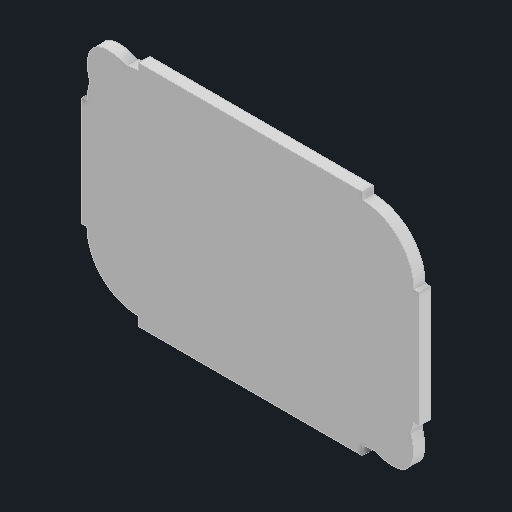
# Autodesk Inventor part: CalibrationTarget
Saved by Autodesk Inventor 2026 (Build 300175050, 175E)
## iProperties
Created: 2024-11-18
Part Number: CalibrationTarget
Material: Generisch
Document SubType Name: Modeling
Designer: neuhau0004
Density: 1 g/cm^3
Appearance: Vorgabe
Author: neuhau0004
Autodesk Inventor part; units mm, degrees
ref_plane "YZ Plane" through (0, 0, 0) normal (1, 0, 0) x (0, 1, 0)
ref_plane "XZ Plane" through (0, 0, 0) normal (0, 1, 0) x (-1, 0, 0)
ref_plane "XY Plane" through (0, 0, 0) normal (0, 0, 1) x (1, 0, 0)
sketch "Skizze1" plane through (0, 0, 0) normal (0, 0, 1) x (1, 0, 0)
  line L0 (-62.3, -42.85) -> (62.3, -42.85)
  line L1 (62.3, -42.85) -> (62.3, 42.85)
  line L2 (62.3, 42.85) -> (-62.3, 42.85)
  line L3 (-62.3, 42.85) -> (-62.3, -42.85)
  line L4 (-62.3, -42.85) -> (62.3, 42.85) construction
  line L5 (62.3, -42.85) -> (-62.3, 42.85) construction
  line L6 (-62, 42.85) -> (62, 42.85)
  line L7 (64, 40.85) -> (64, -40.85)
  line L8 (62, -42.85) -> (-62, -42.85)
  line L9 (-64, -40.85) -> (-64, 40.85)
  line L10 (-64, 42.85) -> (64, -42.85) construction
  line L11 (64, 42.85) -> (-64, -42.85) construction
  circle A0 centre (-40, 19.85) radius 18.45
  circle A1 centre (0, 19.85) radius 18.45
  circle A2 centre (40, 19.85) radius 18.45
  circle A3 centre (-40, -19.15) radius 18.45
  circle A4 centre (0, -19.15) radius 18.45
  circle A5 centre (40, -19.15) radius 18.45
  arc A6 (64, 40.85) -> (62, 42.85) centre (62, 40.85) ccw
  arc A7 (62, -42.85) -> (64, -40.85) centre (62, -40.85) ccw
  arc A8 (-64, -40.85) -> (-62, -42.85) centre (-62, -40.85) ccw
  arc A9 (-62, 42.85) -> (-64, 40.85) centre (-62, 40.85) ccw
  line L12 (-60.3, 40.85) -> (60.3, 40.85)
  line L13 (60.3, 40.85) -> (60.3, -40.85)
  line L14 (60.3, -40.85) -> (-60.3, -40.85)
  line L15 (-60.3, -40.85) -> (-60.3, 40.85)
  line L16 (-60.3, 40.85) -> (60.3, -40.85) construction
  line L17 (60.3, 40.85) -> (-60.3, -40.85) construction
  ellipse E0 centre (40, 19.85) end of major axis (24, 37.55) minor radius 11.9962
  ellipse E1 centre (0, 19.85) end of major axis (-16, 37.55) minor radius 11.9962
  ellipse E2 centre (-40, 19.85) end of major axis (-56, 37.55) minor radius 11.9962
  ellipse E3 centre (40, -19.15) end of major axis (24, -1.45) minor radius 11.9962
  ellipse E4 centre (0, -19.15) end of major axis (-16, -1.45) minor radius 11.9962
  ellipse E5 centre (-40, -19.15) end of major axis (-56, -1.45) minor radius 11.9962
  line L18 (-40, 40.85) -> (-60.3, 40.85)
  line L19 (-60.3, 40.85) -> (-60.3, 19.85)
  line L20 (-58.45, 19.85) -> (-60.3, 19.85)
  line L21 (-58.45, -19.15) -> (-60.3, -19.15)
  line L22 (-60.3, -40.85) -> (-60.3, -19.15)
  line L23 (-40, -37.6) -> (-40, -40.85)
  line L24 (-60.3, -40.85) -> (-40, -40.85)
  arc A10 (-40, 38.3) -> (-58.45, 19.85) centre (-40, 19.85) ccw
  line L25 (-40, 40.85) -> (-40, 38.3)
  line L26 (40, 38.3) -> (40, 40.85)
  line L27 (58.45, 19.85) -> (60.3, 19.85)
  line L28 (58.45, -19.15) -> (60.3, -19.15)
  line L29 (40, -37.6) -> (40, -40.85)
  line L30 (-60.3, -19.15) -> (-60.3, -21.55)
  line L31 (-60.3, -21.55) -> (-58.2932, -21.55)
  line L32 (60.3, -21.55) -> (58.2932, -21.55)
  point P0 (0, 0)
  point P1 (0, 0)
  point P2 (62, 42.85)
  point P3 (-22.5977, -25.2789)
  point P4 (-35.6534, -37.0807)
  point P5 (-57.4023, -13.0211)
  point P6 (-44.3466, -1.2193)
  point P7 (17.4023, -25.2789)
  point P8 (4.3466, -37.0807)
  point P9 (-17.4023, -13.0211)
  point P10 (-4.3466, -1.2193)
  point P11 (57.4023, -25.2789)
  point P12 (44.3466, -37.0807)
  point P13 (22.5977, -13.0211)
  point P14 (35.6534, -1.2193)
  point P15 (-22.5977, 13.7211)
  point P16 (-35.6534, 1.9193)
  point P17 (-57.4023, 25.9789)
  point P18 (-44.3466, 37.7807)
  point P19 (17.4023, 13.7211)
  point P20 (4.3466, 1.9193)
  point P21 (-17.4023, 25.9789)
  point P22 (-4.3466, 37.7807)
  point P23 (57.4023, 13.7211)
  point P24 (44.3466, 1.9193)
  point P25 (22.5977, 25.9789)
  point P26 (35.6534, 37.7807)
  point P27 (17.4023, -25.2789)
  point P28 (4.3466, -37.0807)
  point P29 (-17.4023, -13.0211)
  point P30 (-4.3466, -1.2193)
  point P31 (22.5977, -13.0211)
  point P32 (35.6534, -1.2193)
  point P33 (57.4023, 13.7211)
  point P34 (44.3466, 1.9193)
  point P35 (22.5977, 25.9789)
  point P36 (35.6534, 37.7807)
  point P37 (-22.5977, 13.7211)
  point P38 (-35.6534, 1.9193)
  point P39 (-57.4023, -13.0211)
  point P40 (-44.3466, -1.2193)
  point P41 (-22.5977, -25.2789)
  point P42 (-35.6534, -37.0807)
  point P43 (17.4023, 13.7211)
  point P44 (4.3466, 1.9193)
  point P45 (-17.4023, 25.9789)
  point P46 (-4.3466, 37.7807)
  point P47 (-62.3, 42.8274)
  point P48 (-62.3, -42.8274)
  point P49 (-44.3466, 37.7807)
  point P50 (-57.4023, 25.9789)
  point P51 (62.3, -42.8274)
  point P52 (44.3466, -37.0807)
  point P53 (57.4023, -25.2789)
  point P54 (62, 42.85)
  point P55 (62.3, 42.8274)
  dimension "d8" = 124.6
  dimension "d9" = 85.7
  dimension "d10" = 128
  dimension "d11" = 85.7
  dimension "d12" = 36.9
  dimension "d13" = 22.3
  dimension "d14" = 40
  dimension "d15" = 39
  dimension "d16" = 23
  dimension "d17" = 2
  dimension "d18" = 2
  dimension "d19" = 120.6
  dimension "d20" = 81.7
  dimension "d21" = 40
  dimension "d22" = 39
  dimension "d23" = 2.4
  constraints: 66 end point, 20 point on circle, 18 point on line, 13 perpendicular, 11 centre point, 8 tangent, 7 horizontal, 6 midpoint, 6 parallel, 6 vertical, 2 coincident, 2 collinear, 2 equal radius, 27 other
  measures "d8" distance of L2.end L1.end
  measures "d9" distance of L1.end L0.end
  measures "d10" distance of L10.end L11.end
  measures "d11" distance of L11.start L10.end
  measures "d12" diameter of A0
  measures "d13" distance from line of L3 A0.centre
  measures "d14" distance of A0.centre A1.centre
  measures "d15" distance of A0.centre A3.centre
  measures "d16" distance from line of L2 A0.centre
  measures "d17" radius of A6
  measures "d18" radius of A8
  measures "d19" distance of L13.end L14.end
  measures "d20" distance of L12.end L13.end
  measures "d21" distance of point (40, 19.85) point (0, 19.85)
  measures "d22" distance of point (40, 19.85) point (40, -19.15)
  measures "d23" distance of L21.end L30.end
extrude "Extrusion1" add sketch "Skizze1" along normal blind 4 contours A0 E2 | A0 L25 L12 L26 A2 E0 L27 L13 L28 A5 E3 L29 L14 L23 A3 E5 L21 L15 L20 E2 | E2 A0 | A0 E2 | A0 E2 | A0 E2 | A2 E0 | E0 A2 | A2 E0 | A3 E5 | L13 L32 A5 L28 | E0 A2 | E0 A2 | E5 A3 | A3 E5 | A5 E3 | A3 E5 | A3 E5 | E3 A5 | A5 E3 | E3 A5 | E3 A5 | A1 E1 | E1 A1 | A1 E1 | E1 A1 | E1 A1 | A4 E4 | E4 A4 | A4 E4 | E4 A4 | E4 A4
